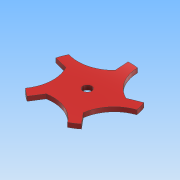
# Autodesk Inventor part: Timing_Star
Saved by Autodesk Inventor 2018.1 (Build 221171000, 171)
## iProperties
Created: 2019-02-11
Part Number: Timing_Star
Material: Generic
Document SubType Name: Modeling
Designer: James
Density: 1 g/cm^3
Appearance: Default
Mass: 3.91056 g
Surface Area: 32.4947 cm^2
Volume: 3.91056 cm^3
Author: James
Autodesk Inventor part; units mm, degrees
ref_plane "YZ Plane" through (0, 0, 0) normal (1, 0, 0) x (0, 1, 0)
ref_plane "XZ Plane" through (0, 0, 0) normal (0, 1, 0) x (-1, 0, 0)
ref_plane "XY Plane" through (0, 0, 0) normal (0, 0, 1) x (1, 0, 0)
sketch "Sketch1" plane through (0, 0, 0) normal (0, 0, 1) x (1, 0, 0)
  circle A0 centre (0, 0) radius 30
  dimension "d0" = 60
  constraints: 1 centre point, 1 coincident
  measures "d0" diameter of A0
extrude "Extrusion1" add sketch "Sketch1" along normal blind 3
sketch "Sketch2" plane through (0, 0, 3) normal (0, 0, 1) x (1, 0, 0)
  circle A0 centre (0, 0) radius 30 projected
  circle A1 centre (30, 30) radius 25
  dimension "d6" = 50
  dimension "d7" = 30
  dimension "d8" = 30
  constraints: 1 centre point
  measures "d6" diameter of A1
  measures "d7" horizontal distance of point (0, 0) A1.centre
  measures "d8" horizontal distance of A1.centre point (0, 0)
extrude "Extrusion2" cut sketch "Sketch2" against normal through all contours A1 A0 | A0 A1 picked at (18.8229, 17.5315) picked at (30.2504, 29.5845)
pattern_circular "Circular Pattern1" count 5 over 360 about axis through (0, 0, -10) along (0, 0, 1) of "Extrusion2"
sketch "Sketch3" plane through (0, 0, 3) normal (0, 0, 1) x (1, 0, 0)
  point P0 (0, 0)
  point P1 (0, 0)
  constraints: 1 coincident
hole "Hole1" at (0, 0, 3) direction (0, 0, -1) diameter 6 end through all
sketch "Sketch5" plane through (0, 0, 3) normal (0, 0, 1) x (1, 0, 0)
  arc A0 (4.382, 29.6782) -> (-1.8842, 29.9408) centre (0, 0) ccw
  arc A1 (2.9897, 20.2485) -> (-1.2855, 20.4276) centre (0, 0) ccw
  line L0 (0, 0) -> (-1.8842, 29.9408) construction
  line L1 (0, 0) -> (4.382, 29.6782) construction
  circle A2 centre (0, 0) radius 3 construction
  arc A3 (29.6782, 4.382) -> (13.8993, -26.5859) centre (37.8022, -19.2612) ccw construction
  arc A4 (29.6782, 4.382) -> (29.5798, 5.0035) centre (0, 0) ccw construction
  arc A5 (5.0035, 29.5798) -> (29.5798, 5.0035) centre (30, 30) ccw construction
  arc A6 (5.0035, 29.5798) -> (4.382, 29.6782) centre (0, 0) ccw construction
  arc A7 (-26.5859, 13.8993) -> (4.382, 29.6782) centre (-19.2612, 37.8022) ccw construction
  arc A8 (-26.5859, 13.8993) -> (-26.8716, 13.3386) centre (0, 0) ccw construction
  arc A9 (-21.4345, -20.9896) -> (-26.8716, 13.3386) centre (-41.9041, -6.637) ccw construction
  arc A10 (-21.4345, -20.9896) -> (-20.9896, -21.4345) centre (0, 0) ccw construction
  arc A11 (13.3386, -26.8716) -> (-20.9896, -21.4345) centre (-6.637, -41.9041) ccw construction
  arc A12 (13.3386, -26.8716) -> (13.8993, -26.5859) centre (0, 0) ccw construction
  arc A13 (5.0035, 29.5798) -> (29.5798, 5.0035) centre (30, 30) ccw construction
  line L2 (-1.2855, 20.4276) -> (-1.8842, 29.9408)
  line L3 (4.382, 29.6782) -> (2.9897, 20.2485)
  arc A14 (-26.5859, 13.8993) -> (4.382, 29.6782) centre (-19.2612, 37.8022) ccw projected
  dimension "d28" = 12
  constraints: 8 end point, 5 point on circle, 2 centre point, 2 coincident, 2 point on line
  measures "d28" angle of L1 L0
extrude "Extrusion3" add sketch "Sketch5" against normal up to surface (3 mm away)
pattern_circular "Circular Pattern2" count 5 over 360 about axis through (0, 0, -10) along (0, 0, 1) of "Extrusion3"
equation "\"d8\" = d7"
body "Solid1"
